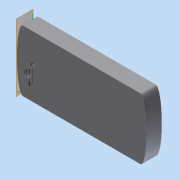
# Autodesk Inventor part: SprintSamsungGalaxyS
Saved by Autodesk Inventor 2011 SP1 (Build 150282100, 282)
## iProperties
Created: 2011-08-14
Part Number: SprintSamsungGalaxyS
Document SubType Name: Modeling
Designer: dgitz
Density: 1 g/cm^3
Author: dgitz
Autodesk Inventor part; units mm, degrees
ref_plane "XZ Plane" through (0, 0, 0) normal (0, 1, 0) x (-1, 0, 0)
ref_plane "XY Plane" through (0, 0, 0) normal (0, 0, 1) x (1, 0, 0)
sketch "Sketch1" plane through (0, 0, 0) normal (0, 0, 1) x (1, 0, 0)
  line L0 (-62.23, 32.385) -> (62.23, 32.385)
  line L1 (62.23, -32.385) -> (-62.23, -32.385)
  line L2 (62.23, 0) -> (68.58, 0) construction
  line L3 (-62.23, 0) -> (-68.58, 0) construction
  ellipse E0 centre (-62.23, 0) end of major axis (-68.58, 0) minor radius 32.385 (-62.23, 32.385) -> (-62.23, -32.385) ccw
  ellipse E1 centre (62.23, 0) end of major axis (68.58, 0) minor radius 32.385 (62.23, -32.385) -> (62.23, 32.385) ccw
  point P0 (0, 0)
  dimension "d2" = 64.77
  dimension "d3" = 32.385
  dimension "d4" = 6.35
  dimension "d5" = 6.35
  dimension "d6" = 62.23
  dimension "d7" = 68.58
  constraints: 8 end point, 7 horizontal, 2 coincident, 2 parallel, 1 collinear, 10 other
  measures "d2" distance between parallel lines of L1 L0
  measures "d3" distance from line of point (0, 0) L0
  measures "d4" distance of L2.start L2.end
  measures "d5" distance of L3.start L3.end
  measures "d6" distance of point (0, 0) point (-62.23, 0)
  measures "d7" distance of L2.end point (0, 0)
extrude "Extrusion1" add sketch "Sketch1" along normal blind 16.256
ref_plane "Work Plane1" through (-68.58, 0, 0) normal (1, 0, 0) x (0, 1, 0)
sketch "Sketch2" plane through (0, 0, 0) normal (1, 0, 0) x (0, 1, 0)
  point P0 (0, 0)
sketch "Sketch3" plane through (-68.58, 0, 0) normal (1, 0, 0) x (0, 1, 0)
  circle A0 centre (-15.5448, 4.1402) radius 1.6002
  line L0 (-32.385, 0) -> (32.385, 0) projected
  line L1 (-32.385, 0) -> (-32.385, 16.256) projected
  point P0 (0, 0)
  dimension "d10" = 3.2004
  dimension "d11" = 2.54
  dimension "d12" = 15.24
  constraints: 1 centre point
  measures "d10" diameter of A0
  measures "d11" distance edge to line of A0 L0
  measures "d12" distance edge to line of A0 L1
body "Solid1"
